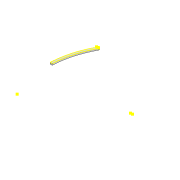
# Autodesk Inventor part: Part_13_p2
Saved by Autodesk Inventor 2022 (Build 260153000, 153)
## iProperties
Created: 2022-04-26
Part Number: Part_13_p2
Material: Generic
Document SubType Name: Modeling
Designer: dell
Density: 1 g/cm^3
Appearance: Default
Author: dell
Autodesk Inventor part; units mm, degrees
ref_plane "YZ Plane" through (0, 0, 0) normal (1, 0, 0) x (0, 1, 0)
ref_plane "XZ Plane" through (0, 0, 0) normal (0, 1, 0) x (-1, 0, 0)
ref_plane "XY Plane" through (0, 0, 0) normal (0, 0, 1) x (1, 0, 0)
sketch "Sketch1" plane through (0, 0, 0) normal (0, 1, 0) x (-1, 0, 0)
  line L0 (0, 0) -> (0, -382.775) construction
  line L1 (-5, 0) -> (-5, -382.775)
  line L2 (5, -382.775) -> (5, 0)
  arc A0 (5, 0) -> (-5, 0) centre (0, 0) ccw
  arc A1 (-5, -382.775) -> (5, -382.775) centre (0, -382.775) ccw
  circle A2 centre (0, 0) radius 1.5
  circle A3 centre (0, -382.775) radius 1.5
  arc A4 (5, -382.775) -> (5, 0) centre (-346.2418, -191.3875) ccw
  arc A5 (-5, -382.775) -> (-5, 0) centre (-356.2418, -191.3875) ccw
  point P0 (0, -191.3875)
  dimension "d0" = 382.775
  dimension "d1" = 10
  dimension "d2" = 3
  dimension "d3" = 3
  dimension "d12" = 400
  dimension "d13" = 400
  constraints: 8 end point, 8 point on circle, 6 centre point, 4 tangent, 2 coincident, 1 midpoint, 1 parallel, 1 vertical
  measures "d0" distance of L0.start L0.end
  measures "d1" diameter of A1
  measures "d2" diameter of A2
  measures "d3" diameter of A3
  measures "d12" radius of A4
  measures "d13" radius of A5
extrude "Extrusion1" add sketch "Sketch1" along normal blind 8 contours A0 L2 A5 | A5 L2 A1 | A4 L2 A5
fillet "Fillet1" radius 2 4 edges at (5, 4, -382.775) (-5, 4, -382.775) (-5, 4, 0) (5, 4, 0)
sketch "Sketch2" plane through (0, 0, 0) normal (0, -1, 0) x (1, 0, 0)
  arc A0 (-4.9846, -383.1668) -> (4.9441, -383.5202) centre (0, -382.775) ccw projected
  arc A1 (4.9441, 0.7452) -> (-4.9846, 0.3918) centre (0, 0) ccw projected
  circle A2 centre (0, -382.775) radius 1.5 projected
  circle A3 centre (0, 0) radius 1.5 projected
  arc A4 (-5.2212, -0.4065) -> (-5.2212, -382.3685) centre (346.2418, -191.3875) ccw projected
  arc A5 (4.7241, -0.5073) -> (4.7241, -382.2677) centre (356.2418, -191.3875) ccw projected
  arc A6 (4.7241, -0.5073) -> (4.9441, 0.7452) centre (2.9665, 0.4471) ccw projected
  arc A7 (-5.2212, -0.4065) -> (-4.9846, 0.3918) centre (-6.9785, 0.5485) ccw projected
  arc A8 (-4.9846, -383.1668) -> (-5.2212, -382.3685) centre (-6.9785, -383.3235) ccw projected
  arc A9 (4.9441, -383.5202) -> (4.7241, -382.2677) centre (2.9665, -383.2221) ccw projected
sketch "Sketch3" plane through (0, 8, 0) normal (0, 1, 0) x (1, 0, 0)
  line L0 (-111.727, 425.5197) -> (93.4733, 425.5197)
  line L1 (93.4733, 425.5197) -> (93.4733, -68.38)
  line L2 (93.4733, -68.38) -> (-111.727, -68.38)
  line L3 (-111.727, -68.38) -> (-111.727, 425.5197)
  line L4 (-64.7929, 400.3549) -> (33.9871, 400.3549)
  line L5 (33.9871, 400.3549) -> (33.9871, 210)
  line L6 (33.9871, 210) -> (-64.7929, 210)
  line L7 (-64.7929, 210) -> (-64.7929, 400.3549)
  line L8 (-64.7929, 210) -> (33.9871, 210)
  line L9 (33.9871, 210) -> (33.9871, 30)
  line L10 (33.9871, 30) -> (-64.7929, 30)
  line L11 (-64.7929, 30) -> (-64.7929, 210)
  point P0 (0, 0)
  dimension "d15" = 30
  dimension "d16" = 180
  dimension "d17" = 190.3549
  constraints: 24 end point, 6 parallel, 3 horizontal, 3 perpendicular
  measures "d15" distance from line of L10 point (0, 0)
  measures "d16" distance of L8.end L9.end
  measures "d17" distance of L4.end L5.end
extrude "Extrusion2" cut sketch "Sketch3" along normal mid plane 20 contours L0 L1 L2 L3 | L6 L9 L10 L11
sketch "Sketch4" plane through (0, 8, 0) normal (0, 1, 0) x (1, 0, 0)
  circle A0 centre (0, 382.775) radius 1.5 projected
  line L0 (-53.3249, 210) -> (-43.3249, 210) projected
  arc A1 (4.7241, 382.2677) -> (-43.3249, 210) centre (356.2418, 191.3875) ccw projected
  arc A2 (4.7241, 382.2677) -> (4.9441, 383.5202) centre (2.9665, 383.2221) ccw projected
  arc A3 (4.9441, 383.5202) -> (-4.9846, 383.1668) centre (0, 382.775) ccw projected
  arc A4 (-5.2212, 382.3685) -> (-4.9846, 383.1668) centre (-6.9785, 383.3235) ccw projected
  arc A5 (-5.2212, 382.3685) -> (-53.3249, 210) centre (346.2418, 191.3875) ccw projected
  point P0 (0, 0)
body "Solid1"
